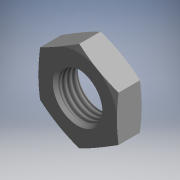
# Autodesk Inventor part: DIN-439-B - M12x1.25(F)
Saved by Autodesk Inventor 2017.3 (Build 213256000, 256)
## iProperties
Part Number: DIN-439-B - M12x1.25(F)
Material: Generic
Catalog Web Link: www.cadenas.de
Description: DIN-439 Form B-Hex nut
Vendor: FESTO
Document SubType Name: Modeling
Designer: partserver
Manufacturer: FESTO
Mass: 1.31793 g
Surface Area: 10.0021 cm^2
Volume: 1.31793 cm^3
Density: 1 g/cm^3
Appearance: PSOLRGB-192-192-192
Category: PARTsolutions
Company: FESTO
Title: DIN-439-B - M12x1.25
Author: Cadenas PARTsolutions
Comments: Hex nut
PSOL_IDENT_0: {$CADENAS_DATA\23d-libs\festo\zyl_zubeh\din_439_b\din_439_form_b.prj},192 {VTYP=3D},{NB=DIN-439-B -
PSOL_IDENT_1: M12x1.25(F)},{LINA=DIN-439-B - M12x1.25},{NN=DIN-439 Form B},{DATE=28.05.2015 11:05:12},{GEOMDATE=28
PSOL_IDENT_2: .05.2015 08:07:00},{VERSION=},{LINEID=150},{WBVAR=},{WBNUMERIC=}  {NB=DIN-439-B - M12x1.25(F)},{LINA=
PSOL_IDENT_3: DIN-439-B - M12x1.25},{KT=X},{IDNR=},{NENN=M12x1.25},{DG=12.000},{DK=10.647},{M=6.000},{S=19.000},{P=
PSOL_IDENT_4: 1.250}
NB: DIN-439-B - M12x1.25(F)
NN: DIN-439 Form B
NT: Hex nut
NBSYN: DIN-439-B - $NENN.(F)
LINA: DIN-439-B - M12x1.25
CATALOG: Festo
ROWDESC: M12x1.25
NENN: M12x1.25
DG: 12
DK: 10.647
M: 6
S: 19
P: 1.25
SUPPLIER: FESTO
ARTICLENO: DIN-439-B - M12x1.25(F)
BOMINFO: DIN-439-B - M12x1.25
CREATOR: CADENAS GmbH
Autodesk Inventor part; units mm, degrees
sketch "Sketch_1" plane through (0, 0, 0) normal (0, 0, 1) x (1, 0, 0)
  line L0 (0, -6) -> (0, 0)
  line L1 (0, 0) -> (9.45, 0)
  line L2 (9.45, 0) -> (20.6462, -3)
  line L3 (20.6462, -3) -> (9.45, -6)
  line L4 (9.45, -6) -> (0, -6)
  line L5 (0, -6) -> (0, 0)
  constraints: 12 end point
revolve "Revolution1" add sketch "Sketch_1" angle 360 about axis through (0, -6, 0) along (0, 1, 0)
sketch "Sketch_2" plane through (0, 0, 0) normal (0, 1, 0) x (-1, 0, 0)
  line L0 (38, -38) -> (38, 38)
  line L1 (38, 38) -> (-38, 38)
  line L2 (-38, 38) -> (-38, -38)
  line L3 (-38, -38) -> (38, -38)
  line L4 (9.5, 5.4848) -> (0, 10.9697)
  line L5 (0, 10.9697) -> (-9.5, 5.4848)
  line L6 (-9.5, 5.4848) -> (-9.5, -5.4848)
  line L7 (-9.5, -5.4848) -> (0, -10.9697)
  line L8 (0, -10.9697) -> (9.5, -5.4848)
  line L9 (9.5, -5.4848) -> (9.5, 5.4848)
  constraints: 20 end point
extrude "Extrusion1" cut sketch "Sketch_2" along normal mid plane 14
sketch "Sketch_3" plane through (0, 0, 0) normal (0, 0, 1) x (1, 0, 0)
  line L0 (0, -6) -> (0, 0)
  line L1 (0, 0) -> (6, 0)
  line L2 (6, 0) -> (5.3235, -0.6765)
  line L3 (5.3235, -0.6765) -> (5.3235, -5.3235)
  line L4 (5.3235, -5.3235) -> (6, -6)
  line L5 (6, -6) -> (0, -6)
  line L6 (0, -6) -> (0, 0)
  constraints: 14 end point
revolve "Revolution2" cut sketch "Sketch_3" angle 360 about axis through (0, -6, 0) along (0, -1, 0)
thread "Thread1" size "M12x1.25" class "6H" standard "ISO Metric profile" full length
ref_plane "2CYL_XY" through (0, -3, 0) normal (0, 1, 0) x (1, 0, 0)
ref_plane "2CYL_YZ" through (0, -3, 0) normal (1, 0, 0) x (0, 0, -1)
ref_plane "2CYL_ZX" through (0, -3, 0) normal (0, 0, -1) x (0, 1, 0)
ref_plane "din439b_punkt_XY" through (0, 0, 0) normal (0, 1, 0) x (1, 0, 0)
ref_plane "din439b_punkt_YZ" through (0, 0, 0) normal (1, 0, 0) x (0, 0, -1)
ref_plane "din439b_punkt_ZX" through (0, 0, 0) normal (0, 0, -1) x (0, 1, 0)
body "Solid1"
